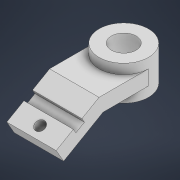
# Autodesk Inventor part: Pieza de practica 14
Saved by Autodesk Inventor 2022 (Build 260153000, 153)
## iProperties
Created: 2022-09-27
Part Number: Pieza de practica 14
Material: Genérico
Document SubType Name: Modeling
Designer: aleon
Density: 1 g/cm^3
Appearance: Valor por defecto
Author: aleon
Autodesk Inventor part; units mm, degrees
ref_plane "YZ Plane" through (0, 0, 0) normal (1, 0, 0) x (0, 1, 0)
ref_plane "XZ Plane" through (0, 0, 0) normal (0, 1, 0) x (-1, 0, 0)
ref_plane "XY Plane" through (0, 0, 0) normal (0, 0, 1) x (1, 0, 0)
sketch "Boceto1" plane through (0, 0, 0) normal (1, 0, 0) x (0, 1, 0)
  line L0 (-17.5, -25) -> (17.5, -25)
  line L1 (17.5, -25) -> (17.5, 25)
  line L2 (17.5, 25) -> (-17.5, 25)
  line L3 (-17.5, 25) -> (-17.5, -25)
  line L4 (7.5, 25) -> (7.5, 50)
  line L5 (-7.5, 45.9808) -> (-7.5, 25)
  line L6 (17.5, 12.5) -> (-17.5, 12.5)
  line L7 (17.5, -12.5) -> (-17.5, -12.5)
  line L8 (7.5, 50) -> (-17.5, 93.3013)
  line L9 (-17.5, 93.3013) -> (-30.4904, 85.8013)
  line L10 (-30.4904, 85.8013) -> (-7.5, 45.9808)
  line L11 (-40.0885, 0) -> (27.0981, 0) projected
  point P0 (0, 0)
  dimension "d0" = 10
  dimension "d1" = 10
  dimension "d2" = 15
  dimension "d3" = 25
  dimension "d5" = 12.5
  dimension "d6" = 50
  dimension "d7" = 12.5
  dimension "d8" = 7.5
  dimension "d9" = 25
  dimension "d10" = 50
  dimension "d11" = 15
  dimension "d12" = 150
  constraints: 22 end point, 6 perpendicular, 6 point on line, 2 parallel, 1 horizontal, 1 vertical
  measures "d0" horizontal distance of L4.start L0.end
  measures "d1" horizontal distance of L0.start L5.end
  measures "d2" distance of L5.end L4.start
  measures "d3" distance between parallel lines of L7 L6
  measures "d5" distance of L7.end L0.start
  measures "d6" distance of L1.end L0.end
  measures "d7" distance from line of L7 point (0, 0)
  measures "d8" horizontal distance of L4.start point (0, 0)
  measures "d9" distance of L4.end L4.start
  measures "d10" distance of L4.end L8.end
  measures "d11" distance of L8.end L9.end
  measures "d12" angle of L5 L10
revolve "Revolución1" add sketch "Boceto1" angle 360 about axis through (0, -10, 0) along (0, 1, 0) contours L3 L2 L1 L6
extrude "Extrusión1" add sketch "Boceto1" along normal mid plane 50 contours L5 L10 L9 L8 L4 L2
sketch "Boceto2" plane through (25, 7.5, 25) normal (0, 0, -1) x (-1, 0, 0)
  line L0 (25, -15) -> (25, 0) projected
  line L1 (25, 0) -> (0, 0) projected
  line L2 (0, -15) -> (0, 0) projected
  line L3 (25, -15) -> (0, -15) projected
  line L4 (50, -15) -> (25, -15) projected
  line L5 (50, 0) -> (50, -15) projected
  line L6 (50, 0) -> (25, 0) projected
  point P0 (25, -7.5)
extrude "Extrusión2" add sketch "Boceto2" along normal up to surface
sketch "Boceto3" plane through (-25, -17.5, 93.3013) normal (0, 0.866, 0.5) x (1, 0, 0)
  line L0 (0, 0) -> (0, 50) projected
  line L1 (0, 30) -> (50, 30)
  line L2 (50, 30) -> (50, 20)
  line L3 (50, 0) -> (50, 45.9808) projected
  line L4 (0, 30) -> (0, 20)
  line L5 (50, 20) -> (0, 20)
  line L6 (0, 50) -> (50, 50) projected
  circle A0 centre (25, 10) radius 5
  point P0 (25, 89.5513)
  point P1 (0, 25)
  dimension "d18" = 10
  dimension "d19" = 5
  dimension "d20" = 25
  dimension "d21" = 10
  dimension "d22" = 10
  constraints: 8 end point, 3 point on line, 1 centre point, 1 horizontal, 1 midpoint, 1 perpendicular
  measures "d18" distance between parallel lines of L5 L1
  measures "d19" distance of point (0, 25) L1.start
  measures "d20" distance from line of point (0, 25) L6
  measures "d21" diameter of A0
  measures "d22" distance from line of L5 A0.centre
extrude "Extrusión3" cut sketch "Boceto3" against normal blind 5 contours L0 L1 L2 L5
extrude "Extrusión4" cut sketch "Boceto3" against normal through all contours A0
